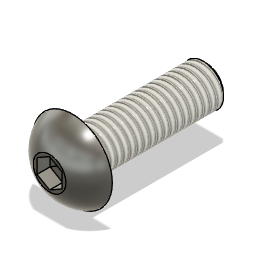
Microstat  Assembly v9 (Autodesk Fusion 360 archive; units mm, degrees)
design "Broached Hexagon Socket Button Head Cap Screw ASME B18.3.4M - M5 x 0.8 x 16 Steel Grade 2 Plain"
description: Broached Hexagon Socket Button Head Cap Screw ASME B18.3.4M - M5 x 0.8 x 16
part number: BHSBHCS ASME B18.3.4M - M5 x 0.8 x 16 Steel Grade 2 Plain
Autodesk Fusion 360 part; units mm, degrees
sketch "Sketch1" plane through (0, 0, 0) normal (0, 1, 0) x (1, 0, 0)
  line L0 (-2.5, 0) -> (-2.5, 16)
  line L1 (-2.5, 16) -> (0, 16)
  line L2 (0, 16) -> (0, -2.75)
  line L3 (-2.5, 0) -> (-4.75, 0)
  line L4 (0, -2.75) -> (-1.95, -2.75)
  arc A0 (-4.75, 0) -> (-1.95, -2.75) centre (0, 2.0359) ccw
  dimension "d9" = 5
  dimension "d66" = 9.5
  dimension "d98" = 3.9
  dimension "d105" = 2.75
  dimension "d106" = 16
  constraint perpendicular L0 L1
  constraint perpendicular L0 L3
  constraint coincident origin L3
  constraint vertical L0
  constraint vertical L2
  constraint coincident origin L2
  constraint perpendicular L2 L4
  constraint coincident L2 A0.centre
  measures "d105" distance of L3 L4
  measures "d106" distance of origin L1
revolve "Revolve1" add sketch "Sketch1" angle 360 about axis through (0, 0, -16) along (0, 0, 1)
ref_plane "WorkPlane1" through (0, 0, 2.75) normal (0, 0, 1) x (1, 0, 0)
sketch "Sketch6" plane through (0, 0, 2.75) normal (0, 0, 1) x (1, 0, 0)
  line L0 (-1.5, 0) -> (1.5, 0) construction
  line L1 (0, 0) -> (-1.5, 0.866)
  line L2 (-1.5, -0.866) -> (-1.5, 0.866)
  line L3 (-1.5, -0.866) -> (0, 0)
  dimension "d91" = 150
  dimension "d107" = 3
  constraint horizontal L0
  constraint midpoint L1.start L0
  constraint coincident L1.start L3.end
  constraint perpendicular L0 L2
  constraint midpoint L0.start L2
  constraint coincident L1.end L2.end
  measures "d91" angle of L0 L1
  measures "d107" distance of L0.end L2
extrude "Extrude1" cut sketch "Sketch6" against normal blind 1.56
pattern_circular "C-Pattern1" count 6 over 360 about axis through (0, 0, 1.75) along (0, 0, 1) of "Extrude1"
extrude "Extrude2" cut 1 faces at (0, -0.5774, 1.19) along direction (0, 0, -1) blind 1.56 draft -85
fillet "Fillet5" radius 0.2 1 edges at (-2.3308, 0.904, 0)
thread "Thread5" "ANSI Metric M Profile 5.0 M5x0.8 M5x0.8 4g6g" major diameter 4.901 minor diameter 4.007 pitch 0.8 angle 60 resizes the face on face at (-2.4876, 0.2489, -10.7333) from (0, 0, -1.6) to (0, 0, -16)
sketch "Sketch5" plane through (0, 0, 0) normal (0, 1, 0) x (1, 0, 0)
  line L0 (0, 16) -> (0, -2.75)
  line L1 (0, 16) -> (-2.55, 16)
  line L2 (-2.55, 16) -> (-2.55, 15.5092)
  line L3 (-2.55, 15.5092) -> (-2.0092, 16)
  dimension "d108" = 0.4908
  dimension "d109" = 2.0092
  dimension "d110" = 2.55
  constraint coincident L0.start L1.start
  constraint perpendicular L1 L2
  constraint coincident L1 L3.end
  measures "d108" distance of L1 L2.end
  measures "d109" distance of L0 L3.end
  measures "d110" distance of L0 L2
revolve "Revolve2" cut sketch "Sketch5" angle 360 about axis through (0, 0, -16) along (0, 0, 1)
equation "d9 = adsk_nomdia"
equation "adsk_nomlen = 16.00 mm"
equation "adsk_headh = 2.75 mm"
equation "adsk_headdia = 9.50 mm"
equation "adsk_nomdia = 5.00 mm"
equation "adsk_philwidth = 3.00 mm"
equation "d31 = -adsk_phildepth"
equation "adsk_phildepth = 1.56 mm"
equation "d66 = adsk_headdia"
equation "d71 = adsk_headh"
equation "d76 = -adsk_phildepth"
equation "adsk_thrlen = 14.40 mm"
equation "adsk_endpointdia = 4.01848 mm"
equation "adsk_startlen = 0.49076 mm"
equation "d98 = adsk_philwidth * 1.3"
equation "adsk_midfillet = 0.20 mm"
equation "d104 = adsk_midfillet"
equation "d105 = adsk_headh"
equation "d106 = adsk_nomlen"
equation "d107 = adsk_philwidth"
equation "d108 = adsk_startlen"
equation "d109 = adsk_endpointdia / 2"
equation "d110 = adsk_nomdia * 0.51"
equation "d116 = min(adsk_thrlen; adsk_nomlen - adsk_midfillet - 0.001 mm)"

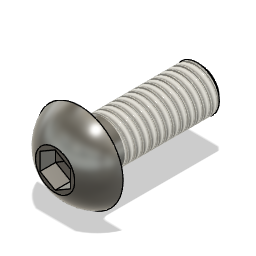
design "Hexagon Socket Button Head Screw ISO 7380-1 - M3 x 8 Steel 4.6 Plain"
description: Hexagon Socket Button Head Screw ISO 7380-1 - M3 x 8
part number: ISO 7380-1 - M3 x 8 Steel 4.6 Plain
Autodesk Fusion 360 part; units mm, degrees
sketch "Sketch1" plane through (0, 0, 0) normal (0, 1, 0) x (1, 0, 0)
  line L0 (-1.5, 0) -> (-1.5, 8)
  line L1 (-1.5, 8) -> (0, 8)
  line L2 (0, 8) -> (0, -1.65)
  line L3 (-1.5, 0) -> (-2.85, 0)
  line L4 (0, -1.65) -> (-1.3, -1.65)
  arc A0 (-2.85, 0) -> (-1.3, -1.65) centre (0, 1.1242) ccw
  dimension "d9" = 3
  dimension "d66" = 5.7
  dimension "d98" = 2.6
  dimension "d105" = 1.65
  dimension "d106" = 8
  constraint perpendicular L0 L1
  constraint perpendicular L0 L3
  constraint coincident origin L3
  constraint vertical L0
  constraint vertical L2
  constraint coincident origin L2
  constraint perpendicular L2 L4
  constraint coincident L2 A0.centre
  measures "d105" distance of L3 L4
  measures "d106" distance of origin L1
revolve "Revolve1" add sketch "Sketch1" angle 360 about axis through (0, 0, -8) along (0, 0, 1)
ref_plane "WorkPlane1" through (0, 0, 1.65) normal (0, 0, 1) x (1, 0, 0)
sketch "Sketch6" plane through (0, 0, 1.65) normal (0, 0, 1) x (1, 0, 0)
  line L0 (-1, 0) -> (1, 0) construction
  line L1 (0, 0) -> (-1, 0.5774)
  line L2 (-1, -0.5774) -> (-1, 0.5774)
  line L3 (-1, -0.5774) -> (0, 0)
  dimension "d91" = 150
  dimension "d107" = 2
  constraint horizontal L0
  constraint midpoint L1.start L0
  constraint coincident L1.start L3.end
  constraint perpendicular L0 L2
  constraint midpoint L0.start L2
  constraint coincident L1.end L2.end
  measures "d91" angle of L0 L1
  measures "d107" distance of L0.end L2
extrude "Extrude1" cut sketch "Sketch6" against normal blind 1.04
pattern_circular "C-Pattern1" count 6 over 360 about axis through (0, 0, 1.75) along (0, 0, 1) of "Extrude1"
extrude "Extrude2" cut 1 faces at (-0.3333, 0.1925, 0.61) along direction (0, 0, -1) blind 1.04 draft -85
fillet "Fillet5" radius 0.3 1 edges at (-1.3985, 0.5424, 0)
thread "Thread5" "ISO Metric profile 3.0 M3x0.5 M3x0.5 6g" major diameter 2.927 minor diameter 2.3555 pitch 0.5 angle 60 resizes the face on face at (-1.4981, 0.0748, -5.4333) from (0, 0, -1.5) to (0, 0, -8)
sketch "Sketch5" plane through (0, 0, 0) normal (0, 1, 0) x (1, 0, 0)
  line L0 (0, 8) -> (0, -1.65)
  line L1 (0, 8) -> (-1.53, 8)
  line L2 (-1.53, 8) -> (-1.53, 7.6933)
  line L3 (-1.53, 7.6933) -> (-1.1933, 8)
  dimension "d108" = 0.3067
  dimension "d109" = 1.1933
  dimension "d110" = 1.53
  constraint coincident L0.start L1.start
  constraint perpendicular L1 L2
  constraint coincident L1 L3.end
  measures "d108" distance of L1 L2.end
  measures "d109" distance of L0 L3.end
  measures "d110" distance of L0 L2
revolve "Revolve2" cut sketch "Sketch5" angle 360 about axis through (0, 0, -8) along (0, 0, 1)
equation "d9 = adsk_nomdia"
equation "adsk_nomlen = 8.00 mm"
equation "adsk_headh = 1.65 mm"
equation "adsk_headdia = 5.70 mm"
equation "adsk_nomdia = 3.00 mm"
equation "adsk_philwidth = 2.00 mm"
equation "d31 = -adsk_phildepth"
equation "adsk_phildepth = 1.04 mm"
equation "d66 = adsk_headdia"
equation "d71 = adsk_headh"
equation "d76 = -adsk_phildepth"
equation "adsk_thrlen = 6.50 mm"
equation "adsk_endpointdia = 2.38655 mm"
equation "adsk_startlen = 0.306725 mm"
equation "d98 = adsk_philwidth * 1.3"
equation "adsk_midfillet = 0.30 mm"
equation "d104 = adsk_midfillet"
equation "d105 = adsk_headh"
equation "d106 = adsk_nomlen"
equation "d107 = adsk_philwidth"
equation "d108 = adsk_startlen"
equation "d109 = adsk_endpointdia / 2"
equation "d110 = adsk_nomdia * 0.51"
equation "d116 = min(adsk_thrlen; adsk_nomlen - adsk_midfillet - 0.001 mm)"

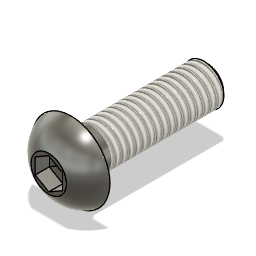
design "Hexagon Socket Button Head Screw ISO 7380-1 - M3 x 10 Steel 4.6 Plain"
description: Hexagon Socket Button Head Screw ISO 7380-1 - M3 x 10
part number: ISO 7380-1 - M3 x 10 Steel 4.6 Plain
Autodesk Fusion 360 part; units mm, degrees
sketch "Sketch1" plane through (0, 0, 0) normal (0, 1, 0) x (1, 0, 0)
  line L0 (-1.5, 0) -> (-1.5, 10)
  line L1 (-1.5, 10) -> (0, 10)
  line L2 (0, 10) -> (0, -1.65)
  line L3 (-1.5, 0) -> (-2.85, 0)
  line L4 (0, -1.65) -> (-1.3, -1.65)
  arc A0 (-2.85, 0) -> (-1.3, -1.65) centre (0, 1.1242) ccw
  dimension "d9" = 3
  dimension "d66" = 5.7
  dimension "d98" = 2.6
  dimension "d105" = 1.65
  dimension "d106" = 10
  constraint perpendicular L0 L1
  constraint perpendicular L0 L3
  constraint coincident origin L3
  constraint vertical L0
  constraint vertical L2
  constraint coincident origin L2
  constraint perpendicular L2 L4
  constraint coincident L2 A0.centre
  measures "d105" distance of L3 L4
  measures "d106" distance of origin L1
revolve "Revolve1" add sketch "Sketch1" angle 360 about axis through (0, 0, -10) along (0, 0, 1)
ref_plane "WorkPlane1" through (0, 0, 1.65) normal (0, 0, 1) x (1, 0, 0)
sketch "Sketch6" plane through (0, 0, 1.65) normal (0, 0, 1) x (1, 0, 0)
  line L0 (-1, 0) -> (1, 0) construction
  line L1 (0, 0) -> (-1, 0.5774)
  line L2 (-1, -0.5774) -> (-1, 0.5774)
  line L3 (-1, -0.5774) -> (0, 0)
  dimension "d91" = 150
  dimension "d107" = 2
  constraint horizontal L0
  constraint midpoint L1.start L0
  constraint coincident L1.start L3.end
  constraint perpendicular L0 L2
  constraint midpoint L0.start L2
  constraint coincident L1.end L2.end
  measures "d91" angle of L0 L1
  measures "d107" distance of L0.end L2
extrude "Extrude1" cut sketch "Sketch6" against normal blind 1.04
pattern_circular "C-Pattern1" count 6 over 360 about axis through (0, 0, 1.75) along (0, 0, 1) of "Extrude1"
extrude "Extrude2" cut 1 faces at (0, 0, 0.61) along direction (0, 0, -1) blind 1.04 draft -85
fillet "Fillet5" radius 0.3 1 edges at (-1.3985, 0.5424, 0)
thread "Thread5" "ISO Metric profile 3.0 M3x0.5 M3x0.5 6g" major diameter 2.927 minor diameter 2.3555 pitch 0.5 angle 60 resizes the face on face at (-1.4981, 0.0748, -6.7667) from (0, 0, -1.5) to (0, 0, -10)
sketch "Sketch5" plane through (0, 0, 0) normal (0, 1, 0) x (1, 0, 0)
  line L0 (0, 10) -> (0, -1.65)
  line L1 (0, 10) -> (-1.53, 10)
  line L2 (-1.53, 10) -> (-1.53, 9.6933)
  line L3 (-1.53, 9.6933) -> (-1.1933, 10)
  dimension "d108" = 0.3067
  dimension "d109" = 1.1933
  dimension "d110" = 1.53
  constraint coincident L0.start L1.start
  constraint perpendicular L1 L2
  constraint coincident L1 L3.end
  measures "d108" distance of L1 L2.end
  measures "d109" distance of L0 L3.end
  measures "d110" distance of L0 L2
revolve "Revolve2" cut sketch "Sketch5" angle 360 about axis through (0, 0, -10) along (0, 0, 1)
equation "d9 = adsk_nomdia"
equation "adsk_nomlen = 10.00 mm"
equation "adsk_headh = 1.65 mm"
equation "adsk_headdia = 5.70 mm"
equation "adsk_nomdia = 3.00 mm"
equation "adsk_philwidth = 2.00 mm"
equation "d31 = -adsk_phildepth"
equation "adsk_phildepth = 1.04 mm"
equation "d66 = adsk_headdia"
equation "d71 = adsk_headh"
equation "d76 = -adsk_phildepth"
equation "adsk_thrlen = 8.50 mm"
equation "adsk_endpointdia = 2.38655 mm"
equation "adsk_startlen = 0.306725 mm"
equation "d98 = adsk_philwidth * 1.3"
equation "adsk_midfillet = 0.30 mm"
equation "d104 = adsk_midfillet"
equation "d105 = adsk_headh"
equation "d106 = adsk_nomlen"
equation "d107 = adsk_philwidth"
equation "d108 = adsk_startlen"
equation "d109 = adsk_endpointdia / 2"
equation "d110 = adsk_nomdia * 0.51"
equation "d116 = min(adsk_thrlen; adsk_nomlen - adsk_midfillet - 0.001 mm)"

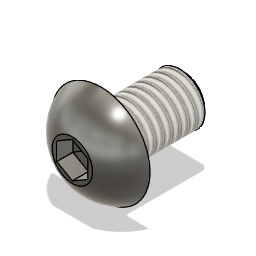
design "Broached Hexagon Socket Button Head Cap Screw ASME B18.3.4M - M5 x 0.8 x 8 Steel Grade 2 Plain"
description: Broached Hexagon Socket Button Head Cap Screw ASME B18.3.4M - M5 x 0.8 x 8
part number: BHSBHCS ASME B18.3.4M - M5 x 0.8 x 8 Steel Grade 2 Plain
Autodesk Fusion 360 part; units mm, degrees
sketch "Sketch1" plane through (0, 0, 0) normal (0, 1, 0) x (1, 0, 0)
  line L0 (-2.5, 0) -> (-2.5, 8)
  line L1 (-2.5, 8) -> (0, 8)
  line L2 (0, 8) -> (0, -2.75)
  line L3 (-2.5, 0) -> (-4.75, 0)
  line L4 (0, -2.75) -> (-1.95, -2.75)
  arc A0 (-4.75, 0) -> (-1.95, -2.75) centre (0, 2.0359) ccw
  dimension "d9" = 5
  dimension "d66" = 9.5
  dimension "d98" = 3.9
  dimension "d105" = 2.75
  dimension "d106" = 8
  constraint perpendicular L0 L1
  constraint perpendicular L0 L3
  constraint coincident origin L3
  constraint vertical L0
  constraint vertical L2
  constraint coincident origin L2
  constraint perpendicular L2 L4
  constraint coincident L2 A0.centre
  measures "d105" distance of L3 L4
  measures "d106" distance of origin L1
revolve "Revolve1" add sketch "Sketch1" angle 360 about axis through (0, 0, -8) along (0, 0, 1)
ref_plane "WorkPlane1" through (0, 0, 2.75) normal (0, 0, 1) x (1, 0, 0)
sketch "Sketch6" plane through (0, 0, 2.75) normal (0, 0, 1) x (1, 0, 0)
  line L0 (-1.5, 0) -> (1.5, 0) construction
  line L1 (0, 0) -> (-1.5, 0.866)
  line L2 (-1.5, -0.866) -> (-1.5, 0.866)
  line L3 (-1.5, -0.866) -> (0, 0)
  dimension "d91" = 150
  dimension "d107" = 3
  constraint horizontal L0
  constraint midpoint L1.start L0
  constraint coincident L1.start L3.end
  constraint perpendicular L0 L2
  constraint midpoint L0.start L2
  constraint coincident L1.end L2.end
  measures "d91" angle of L0 L1
  measures "d107" distance of L0.end L2
extrude "Extrude1" cut sketch "Sketch6" against normal blind 1.56
pattern_circular "C-Pattern1" count 6 over 360 about axis through (0, 0, 1.75) along (0, 0, 1) of "Extrude1"
extrude "Extrude2" cut 1 faces at (0.5, 0.2887, 1.19) along direction (0, 0, -1) blind 1.56 draft -85
fillet "Fillet5" radius 0.2 1 edges at (-2.3308, 0.904, 0)
thread "Thread5" "ANSI Metric M Profile 5.0 M5x0.8 M5x0.8 4g6g" major diameter 4.901 minor diameter 4.007 pitch 0.8 angle 60 resizes the face on face at (-2.4876, 0.2489, -5.4) from (0, 0, -1.6) to (0, 0, -8)
sketch "Sketch5" plane through (0, 0, 0) normal (0, 1, 0) x (1, 0, 0)
  line L0 (0, 8) -> (0, -2.75)
  line L1 (0, 8) -> (-2.55, 8)
  line L2 (-2.55, 8) -> (-2.55, 7.5092)
  line L3 (-2.55, 7.5092) -> (-2.0092, 8)
  dimension "d108" = 0.4908
  dimension "d109" = 2.0092
  dimension "d110" = 2.55
  constraint coincident L0.start L1.start
  constraint perpendicular L1 L2
  constraint coincident L1 L3.end
  measures "d108" distance of L1 L2.end
  measures "d109" distance of L0 L3.end
  measures "d110" distance of L0 L2
revolve "Revolve2" cut sketch "Sketch5" angle 360 about axis through (0, 0, -8) along (0, 0, 1)
equation "d9 = adsk_nomdia"
equation "adsk_nomlen = 8.00 mm"
equation "adsk_headh = 2.75 mm"
equation "adsk_headdia = 9.50 mm"
equation "adsk_nomdia = 5.00 mm"
equation "adsk_philwidth = 3.00 mm"
equation "d31 = -adsk_phildepth"
equation "adsk_phildepth = 1.56 mm"
equation "d66 = adsk_headdia"
equation "d71 = adsk_headh"
equation "d76 = -adsk_phildepth"
equation "adsk_thrlen = 6.40 mm"
equation "adsk_endpointdia = 4.01848 mm"
equation "adsk_startlen = 0.49076 mm"
equation "d98 = adsk_philwidth * 1.3"
equation "adsk_midfillet = 0.20 mm"
equation "d104 = adsk_midfillet"
equation "d105 = adsk_headh"
equation "d106 = adsk_nomlen"
equation "d107 = adsk_philwidth"
equation "d108 = adsk_startlen"
equation "d109 = adsk_endpointdia / 2"
equation "d110 = adsk_nomdia * 0.51"
equation "d116 = min(adsk_thrlen; adsk_nomlen - adsk_midfillet - 0.001 mm)"

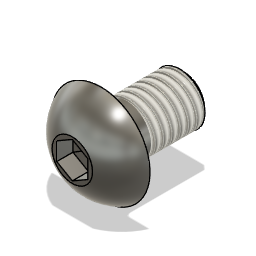
design "Hexagon Socket Button Head Screw ISO 7380-1 - M5 x 8 Steel 4.6 Plain"
description: Hexagon Socket Button Head Screw ISO 7380-1 - M5 x 8
part number: ISO 7380-1 - M5 x 8 Steel 4.6 Plain
Autodesk Fusion 360 part; units mm, degrees
sketch "Sketch1" plane through (0, 0, 0) normal (0, 1, 0) x (1, 0, 0)
  line L0 (-2.5, 0) -> (-2.5, 8)
  line L1 (-2.5, 8) -> (0, 8)
  line L2 (0, 8) -> (0, -2.75)
  line L3 (-2.5, 0) -> (-4.75, 0)
  line L4 (0, -2.75) -> (-1.95, -2.75)
  arc A0 (-4.75, 0) -> (-1.95, -2.75) centre (0, 2.0359) ccw
  dimension "d9" = 5
  dimension "d66" = 9.5
  dimension "d98" = 3.9
  dimension "d105" = 2.75
  dimension "d106" = 8
  constraint perpendicular L0 L1
  constraint perpendicular L0 L3
  constraint coincident origin L3
  constraint vertical L0
  constraint vertical L2
  constraint coincident origin L2
  constraint perpendicular L2 L4
  constraint coincident L2 A0.centre
  measures "d105" distance of L3 L4
  measures "d106" distance of origin L1
revolve "Revolve1" add sketch "Sketch1" angle 360 about axis through (0, 0, -8) along (0, 0, 1)
ref_plane "WorkPlane1" through (0, 0, 2.75) normal (0, 0, 1) x (1, 0, 0)
sketch "Sketch6" plane through (0, 0, 2.75) normal (0, 0, 1) x (1, 0, 0)
  line L0 (-1.5, 0) -> (1.5, 0) construction
  line L1 (0, 0) -> (-1.5, 0.866)
  line L2 (-1.5, -0.866) -> (-1.5, 0.866)
  line L3 (-1.5, -0.866) -> (0, 0)
  dimension "d91" = 150
  dimension "d107" = 3
  constraint horizontal L0
  constraint midpoint L1.start L0
  constraint coincident L1.start L3.end
  constraint perpendicular L0 L2
  constraint midpoint L0.start L2
  constraint coincident L1.end L2.end
  measures "d91" angle of L0 L1
  measures "d107" distance of L0.end L2
extrude "Extrude1" cut sketch "Sketch6" against normal blind 1.56
pattern_circular "C-Pattern1" count 6 over 360 about axis through (0, 0, 1.75) along (0, 0, 1) of "Extrude1"
extrude "Extrude2" cut 1 faces at (0.5, 0.2887, 1.19) along direction (0, 0, -1) blind 1.56 draft -85
fillet "Fillet5" radius 0.45 1 edges at (-2.3308, 0.904, 0)
thread "Thread5" "ISO Metric profile 5.0 M5x0.8 M5x0.8 6g" major diameter 4.901 minor diameter 3.9895 pitch 0.8 angle 60 resizes the face on face at (-2.4876, 0.2489, -5.4833) from (0, 0, -2.4) to (0, 0, -8)
sketch "Sketch5" plane through (0, 0, 0) normal (0, 1, 0) x (1, 0, 0)
  line L0 (0, 8) -> (0, -2.75)
  line L1 (0, 8) -> (-2.55, 8)
  line L2 (-2.55, 8) -> (-2.55, 7.5092)
  line L3 (-2.55, 7.5092) -> (-2.0092, 8)
  dimension "d108" = 0.4908
  dimension "d109" = 2.0092
  dimension "d110" = 2.55
  constraint coincident L0.start L1.start
  constraint perpendicular L1 L2
  constraint coincident L1 L3.end
  measures "d108" distance of L1 L2.end
  measures "d109" distance of L0 L3.end
  measures "d110" distance of L0 L2
revolve "Revolve2" cut sketch "Sketch5" angle 360 about axis through (0, 0, -8) along (0, 0, 1)
equation "d9 = adsk_nomdia"
equation "adsk_nomlen = 8.00 mm"
equation "adsk_headh = 2.75 mm"
equation "adsk_headdia = 9.50 mm"
equation "adsk_nomdia = 5.00 mm"
equation "adsk_philwidth = 3.00 mm"
equation "d31 = -adsk_phildepth"
equation "adsk_phildepth = 1.56 mm"
equation "d66 = adsk_headdia"
equation "d71 = adsk_headh"
equation "d76 = -adsk_phildepth"
equation "adsk_thrlen = 5.60 mm"
equation "adsk_endpointdia = 4.01848 mm"
equation "adsk_startlen = 0.49076 mm"
equation "d98 = adsk_philwidth * 1.3"
equation "adsk_midfillet = 0.45 mm"
equation "d104 = adsk_midfillet"
equation "d105 = adsk_headh"
equation "d106 = adsk_nomlen"
equation "d107 = adsk_philwidth"
equation "d108 = adsk_startlen"
equation "d109 = adsk_endpointdia / 2"
equation "d110 = adsk_nomdia * 0.51"
equation "d116 = min(adsk_thrlen; adsk_nomlen - adsk_midfillet - 0.001 mm)"

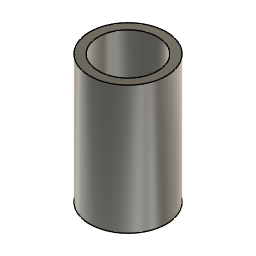
design "inner_payload_rod"
Autodesk Fusion 360 part; units mm, degrees
sketch "Sketch1" plane through (0, 0, 0) normal (0, 0, 1) x (1, 0, 0)
  circle A0 centre (0, 0) radius 7.75
  dimension "d1" = 15.5
  constraint coincident A0.centre origin
  measures "d1" diameter of A0
extrude "Extrude1" add sketch "Sketch1" along normal blind 26
sketch "Sketch2" plane through (0, 0, 26) normal (0, 0, 1) x (-1, 0, 0)
  circle A0 centre (0, 0) radius 7.75
  circle A1 centre (0, 0) radius 6
  dimension "d4" = 12
  constraint concentric A0 A1
  measures "d4" diameter of A1
extrude "Extrude2" cut sketch "Sketch2" against normal blind 26 contours A1

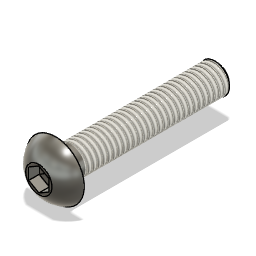
design "Hexagon Socket Button Head Screw ISO 7380-1 - M3 x 16 Steel 4.6 Plain"
description: Hexagon Socket Button Head Screw ISO 7380-1 - M3 x 16
part number: ISO 7380-1 - M3 x 16 Steel 4.6 Plain
Autodesk Fusion 360 part; units mm, degrees
sketch "Sketch1" plane through (0, 0, 0) normal (0, 1, 0) x (1, 0, 0)
  line L0 (-1.5, 0) -> (-1.5, 16)
  line L1 (-1.5, 16) -> (0, 16)
  line L2 (0, 16) -> (0, -1.65)
  line L3 (-1.5, 0) -> (-2.85, 0)
  line L4 (0, -1.65) -> (-1.3, -1.65)
  arc A0 (-2.85, 0) -> (-1.3, -1.65) centre (0, 1.1242) ccw
  dimension "d9" = 3
  dimension "d66" = 5.7
  dimension "d98" = 2.6
  dimension "d105" = 1.65
  dimension "d106" = 16
  constraint perpendicular L0 L1
  constraint perpendicular L0 L3
  constraint coincident origin L3
  constraint vertical L0
  constraint vertical L2
  constraint coincident origin L2
  constraint perpendicular L2 L4
  constraint coincident L2 A0.centre
  measures "d105" distance of L3 L4
  measures "d106" distance of origin L1
revolve "Revolve1" add sketch "Sketch1" angle 360 about axis through (0, 0, -16) along (0, 0, 1)
ref_plane "WorkPlane1" through (0, 0, 1.65) normal (0, 0, 1) x (1, 0, 0)
sketch "Sketch6" plane through (0, 0, 1.65) normal (0, 0, 1) x (1, 0, 0)
  line L0 (-1, 0) -> (1, 0) construction
  line L1 (0, 0) -> (-1, 0.5774)
  line L2 (-1, -0.5774) -> (-1, 0.5774)
  line L3 (-1, -0.5774) -> (0, 0)
  dimension "d91" = 150
  dimension "d107" = 2
  constraint horizontal L0
  constraint midpoint L1.start L0
  constraint coincident L1.start L3.end
  constraint perpendicular L0 L2
  constraint midpoint L0.start L2
  constraint coincident L1.end L2.end
  measures "d91" angle of L0 L1
  measures "d107" distance of L0.end L2
extrude "Extrude1" cut sketch "Sketch6" against normal blind 1.04
pattern_circular "C-Pattern1" count 6 over 360 about axis through (0, 0, 1.75) along (0, 0, 1) of "Extrude1"
extrude "Extrude2" cut 1 faces at (-0.3333, 0.1925, 0.61) along direction (0, 0, -1) blind 1.04 draft -85
fillet "Fillet5" radius 0.3 1 edges at (-1.3985, 0.5424, 0)
thread "Thread5" "ISO Metric profile 3.0 M3x0.5 M3x0.5 6g" major diameter 2.927 minor diameter 2.3555 pitch 0.5 angle 60 resizes the face on face at (-1.4981, 0.0748, -10.7667) from (0, 0, -1.5) to (0, 0, -16)
sketch "Sketch5" plane through (0, 0, 0) normal (0, 1, 0) x (1, 0, 0)
  line L0 (0, 16) -> (0, -1.65)
  line L1 (0, 16) -> (-1.53, 16)
  line L2 (-1.53, 16) -> (-1.53, 15.6933)
  line L3 (-1.53, 15.6933) -> (-1.1933, 16)
  dimension "d108" = 0.3067
  dimension "d109" = 1.1933
  dimension "d110" = 1.53
  constraint coincident L0.start L1.start
  constraint perpendicular L1 L2
  constraint coincident L1 L3.end
  measures "d108" distance of L1 L2.end
  measures "d109" distance of L0 L3.end
  measures "d110" distance of L0 L2
revolve "Revolve2" cut sketch "Sketch5" angle 360 about axis through (0, 0, -16) along (0, 0, 1)
equation "d9 = adsk_nomdia"
equation "adsk_nomlen = 16.00 mm"
equation "adsk_headh = 1.65 mm"
equation "adsk_headdia = 5.70 mm"
equation "adsk_nomdia = 3.00 mm"
equation "adsk_philwidth = 2.00 mm"
equation "d31 = -adsk_phildepth"
equation "adsk_phildepth = 1.04 mm"
equation "d66 = adsk_headdia"
equation "d71 = adsk_headh"
equation "d76 = -adsk_phildepth"
equation "adsk_thrlen = 14.50 mm"
equation "adsk_endpointdia = 2.38655 mm"
equation "adsk_startlen = 0.306725 mm"
equation "d98 = adsk_philwidth * 1.3"
equation "adsk_midfillet = 0.30 mm"
equation "d104 = adsk_midfillet"
equation "d105 = adsk_headh"
equation "d106 = adsk_nomlen"
equation "d107 = adsk_philwidth"
equation "d108 = adsk_startlen"
equation "d109 = adsk_endpointdia / 2"
equation "d110 = adsk_nomdia * 0.51"
equation "d116 = min(adsk_thrlen; adsk_nomlen - adsk_midfillet - 0.001 mm)"

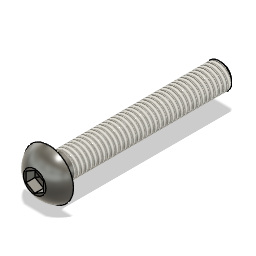
design "Hexagon Socket Button Head Screw ISO 7380-1 - M3 x 20 Steel 4.6 Plain"
description: Hexagon Socket Button Head Screw ISO 7380-1 - M3 x 20
part number: ISO 7380-1 - M3 x 20 Steel 4.6 Plain
Autodesk Fusion 360 part; units mm, degrees
sketch "Sketch1" plane through (0, 0, 0) normal (0, 1, 0) x (1, 0, 0)
  line L0 (-1.5, 0) -> (-1.5, 20)
  line L1 (-1.5, 20) -> (0, 20)
  line L2 (0, 20) -> (0, -1.65)
  line L3 (-1.5, 0) -> (-2.85, 0)
  line L4 (0, -1.65) -> (-1.3, -1.65)
  arc A0 (-2.85, 0) -> (-1.3, -1.65) centre (0, 1.1242) ccw
  dimension "d9" = 3
  dimension "d66" = 5.7
  dimension "d98" = 2.6
  dimension "d105" = 1.65
  dimension "d106" = 20
  constraint perpendicular L0 L1
  constraint perpendicular L0 L3
  constraint coincident origin L3
  constraint vertical L0
  constraint vertical L2
  constraint coincident origin L2
  constraint perpendicular L2 L4
  constraint coincident L2 A0.centre
  measures "d105" distance of L3 L4
  measures "d106" distance of origin L1
revolve "Revolve1" add sketch "Sketch1" angle 360 about axis through (0, 0, -20) along (0, 0, 1)
ref_plane "WorkPlane1" through (0, 0, 1.65) normal (0, 0, 1) x (1, 0, 0)
sketch "Sketch6" plane through (0, 0, 1.65) normal (0, 0, 1) x (1, 0, 0)
  line L0 (-1, 0) -> (1, 0) construction
  line L1 (0, 0) -> (-1, 0.5774)
  line L2 (-1, -0.5774) -> (-1, 0.5774)
  line L3 (-1, -0.5774) -> (0, 0)
  dimension "d91" = 150
  dimension "d107" = 2
  constraint horizontal L0
  constraint midpoint L1.start L0
  constraint coincident L1.start L3.end
  constraint perpendicular L0 L2
  constraint midpoint L0.start L2
  constraint coincident L1.end L2.end
  measures "d91" angle of L0 L1
  measures "d107" distance of L0.end L2
extrude "Extrude1" cut sketch "Sketch6" against normal blind 1.04
pattern_circular "C-Pattern1" count 6 over 360 about axis through (0, 0, 1.75) along (0, 0, 1) of "Extrude1"
extrude "Extrude2" cut 1 faces at (0, 0, 0.61) along direction (0, 0, -1) blind 1.04 draft -85
fillet "Fillet5" radius 0.3 1 edges at (-1.3985, 0.5424, 0)
thread "Thread5" "ISO Metric profile 3.0 M3x0.5 M3x0.5 6g" major diameter 2.927 minor diameter 2.3555 pitch 0.5 angle 60 resizes the face on face at (-1.4981, 0.0748, -13.4333) from (0, 0, -1.5) to (0, 0, -20)
sketch "Sketch5" plane through (0, 0, 0) normal (0, 1, 0) x (1, 0, 0)
  line L0 (0, 20) -> (0, -1.65)
  line L1 (0, 20) -> (-1.53, 20)
  line L2 (-1.53, 20) -> (-1.53, 19.6933)
  line L3 (-1.53, 19.6933) -> (-1.1933, 20)
  dimension "d108" = 0.3067
  dimension "d109" = 1.1933
  dimension "d110" = 1.53
  constraint coincident L0.start L1.start
  constraint perpendicular L1 L2
  constraint coincident L1 L3.end
  measures "d108" distance of L1 L2.end
  measures "d109" distance of L0 L3.end
  measures "d110" distance of L0 L2
revolve "Revolve2" cut sketch "Sketch5" angle 360 about axis through (0, 0, -20) along (0, 0, 1)
equation "d9 = adsk_nomdia"
equation "adsk_nomlen = 20.00 mm"
equation "adsk_headh = 1.65 mm"
equation "adsk_headdia = 5.70 mm"
equation "adsk_nomdia = 3.00 mm"
equation "adsk_philwidth = 2.00 mm"
equation "d31 = -adsk_phildepth"
equation "adsk_phildepth = 1.04 mm"
equation "d66 = adsk_headdia"
equation "d71 = adsk_headh"
equation "d76 = -adsk_phildepth"
equation "adsk_thrlen = 18.50 mm"
equation "adsk_endpointdia = 2.38655 mm"
equation "adsk_startlen = 0.306725 mm"
equation "d98 = adsk_philwidth * 1.3"
equation "adsk_midfillet = 0.30 mm"
equation "d104 = adsk_midfillet"
equation "d105 = adsk_headh"
equation "d106 = adsk_nomlen"
equation "d107 = adsk_philwidth"
equation "d108 = adsk_startlen"
equation "d109 = adsk_endpointdia / 2"
equation "d110 = adsk_nomdia * 0.51"
equation "d116 = min(adsk_thrlen; adsk_nomlen - adsk_midfillet - 0.001 mm)"

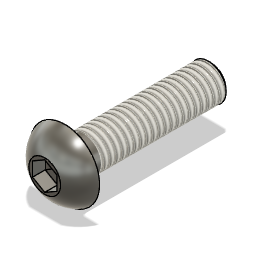
design "Hexagon Socket Button Head Screw ISO 7380-1 - M3 x 12 Steel 4.6 Plain"
description: Hexagon Socket Button Head Screw ISO 7380-1 - M3 x 12
part number: ISO 7380-1 - M3 x 12 Steel 4.6 Plain
Autodesk Fusion 360 part; units mm, degrees
sketch "Sketch1" plane through (0, 0, 0) normal (0, 1, 0) x (1, 0, 0)
  line L0 (-1.5, 0) -> (-1.5, 12)
  line L1 (-1.5, 12) -> (0, 12)
  line L2 (0, 12) -> (0, -1.65)
  line L3 (-1.5, 0) -> (-2.85, 0)
  line L4 (0, -1.65) -> (-1.3, -1.65)
  arc A0 (-2.85, 0) -> (-1.3, -1.65) centre (0, 1.1242) ccw
  dimension "d9" = 3
  dimension "d66" = 5.7
  dimension "d98" = 2.6
  dimension "d105" = 1.65
  dimension "d106" = 12
  constraint perpendicular L0 L1
  constraint perpendicular L0 L3
  constraint coincident origin L3
  constraint vertical L0
  constraint vertical L2
  constraint coincident origin L2
  constraint perpendicular L2 L4
  constraint coincident L2 A0.centre
  measures "d105" distance of L3 L4
  measures "d106" distance of origin L1
revolve "Revolve1" add sketch "Sketch1" angle 360 about axis through (0, 0, -12) along (0, 0, 1)
ref_plane "WorkPlane1" through (0, 0, 1.65) normal (0, 0, 1) x (1, 0, 0)
sketch "Sketch6" plane through (0, 0, 1.65) normal (0, 0, 1) x (1, 0, 0)
  line L0 (-1, 0) -> (1, 0) construction
  line L1 (0, 0) -> (-1, 0.5774)
  line L2 (-1, -0.5774) -> (-1, 0.5774)
  line L3 (-1, -0.5774) -> (0, 0)
  dimension "d91" = 150
  dimension "d107" = 2
  constraint horizontal L0
  constraint midpoint L1.start L0
  constraint coincident L1.start L3.end
  constraint perpendicular L0 L2
  constraint midpoint L0.start L2
  constraint coincident L1.end L2.end
  measures "d91" angle of L0 L1
  measures "d107" distance of L0.end L2
extrude "Extrude1" cut sketch "Sketch6" against normal blind 1.04
pattern_circular "C-Pattern1" count 6 over 360 about axis through (0, 0, 1.75) along (0, 0, 1) of "Extrude1"
extrude "Extrude2" cut 1 faces at (0, 0, 0.61) along direction (0, 0, -1) blind 1.04 draft -85
fillet "Fillet5" radius 0.3 1 edges at (-1.3985, 0.5424, 0)
thread "Thread5" "ISO Metric profile 3.0 M3x0.5 M3x0.5 6g" major diameter 2.927 minor diameter 2.3555 pitch 0.5 angle 60 resizes the face on face at (-1.4981, 0.0748, -8.1) from (0, 0, -1.5) to (0, 0, -12)
sketch "Sketch5" plane through (0, 0, 0) normal (0, 1, 0) x (1, 0, 0)
  line L0 (0, 12) -> (0, -1.65)
  line L1 (0, 12) -> (-1.53, 12)
  line L2 (-1.53, 12) -> (-1.53, 11.6933)
  line L3 (-1.53, 11.6933) -> (-1.1933, 12)
  dimension "d108" = 0.3067
  dimension "d109" = 1.1933
  dimension "d110" = 1.53
  constraint coincident L0.start L1.start
  constraint perpendicular L1 L2
  constraint coincident L1 L3.end
  measures "d108" distance of L1 L2.end
  measures "d109" distance of L0 L3.end
  measures "d110" distance of L0 L2
revolve "Revolve2" cut sketch "Sketch5" angle 360 about axis through (0, 0, -12) along (0, 0, 1)
equation "d9 = adsk_nomdia"
equation "adsk_nomlen = 12.00 mm"
equation "adsk_headh = 1.65 mm"
equation "adsk_headdia = 5.70 mm"
equation "adsk_nomdia = 3.00 mm"
equation "adsk_philwidth = 2.00 mm"
equation "d31 = -adsk_phildepth"
equation "adsk_phildepth = 1.04 mm"
equation "d66 = adsk_headdia"
equation "d71 = adsk_headh"
equation "d76 = -adsk_phildepth"
equation "adsk_thrlen = 10.50 mm"
equation "adsk_endpointdia = 2.38655 mm"
equation "adsk_startlen = 0.306725 mm"
equation "d98 = adsk_philwidth * 1.3"
equation "adsk_midfillet = 0.30 mm"
equation "d104 = adsk_midfillet"
equation "d105 = adsk_headh"
equation "d106 = adsk_nomlen"
equation "d107 = adsk_philwidth"
equation "d108 = adsk_startlen"
equation "d109 = adsk_endpointdia / 2"
equation "d110 = adsk_nomdia * 0.51"
equation "d116 = min(adsk_thrlen; adsk_nomlen - adsk_midfillet - 0.001 mm)"

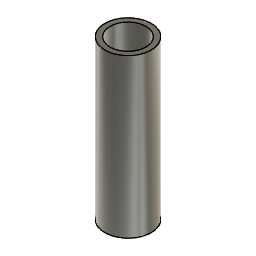
design "payload_chamber_rod"
Autodesk Fusion 360 part; units mm, degrees
sketch "Sketch1" plane through (0, 0, 0) normal (0, 0, 1) x (1, 0, 0)
  circle A0 centre (0, 0) radius 7.75
  dimension "d1" = 15.5
  constraint coincident A0.centre origin
  measures "d1" diameter of A0
extrude "Extrude1" add sketch "Sketch1" along normal blind 27.9
sketch "Sketch2" plane through (0, 0, 27.9) normal (0, 0, 1) x (-1, 0, 0)
  circle A0 centre (0, 0) radius 7.75
  circle A1 centre (0, 0) radius 6
  dimension "d4" = 12
  constraint concentric A0 A1
  measures "d4" diameter of A1
extrude "Extrude2" cut sketch "Sketch2" against normal blind 30 contours A1
extrude "Extrude3" add 1 faces at (7.1155, -0.6831, 27.9) along direction (0, 0, 1) blind 15
extrude "Extrude4" add 1 faces at (7.1155, -0.6831, 42.9) along direction (0, 0, 1) blind 10

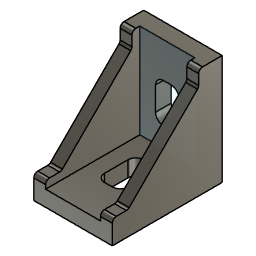
design "Angle Bracket v1"
Autodesk Fusion 360 part; units mm, degrees
sketch "Sketch1" plane through (0, 0, 0) normal (1, 0, 0) x (0, 1, 0)
  line L0 (0, 0) -> (28, 0)
  line L1 (28, 0) -> (28, 28)
  line L2 (28, 28) -> (22, 28)
  line L3 (22, 28) -> (22, 24)
  line L4 (0, 0) -> (0, 6)
  line L5 (0, 6) -> (4, 6)
  line L6 (4, 6) -> (22, 24)
  dimension "d1" = 28
  dimension "d2" = 28
  constraint coincident L0.start L4.start
  constraint horizontal L0
  constraint perpendicular L0 L1
  constraint perpendicular L1 L2
  constraint perpendicular L2 L3
  constraint perpendicular L0 L4
  constraint perpendicular L4 L5
  measures "d1" distance of L0.start L0.end
  measures "d2" distance of L0.end L1.end
extrude "Extrude1" add sketch "Sketch1" along normal blind 3
sketch "Sketch2" plane through (3, 0, 0) normal (1, 0, 0) x (0, 1, 0)
  line L0 (0, 0) -> (28, 0)
  line L1 (28, 0) -> (28, 28)
  line L2 (28, 28) -> (22, 28)
  line L3 (22, 28) -> (22, 24)
  line L4 (22, 24) -> (4, 6)
  line L5 (4, 6) -> (0, 6)
  line L6 (0, 6) -> (0, 0)
  line L7 (0, 0) -> (28, 0)
  line L8 (28, 0) -> (28, 4)
  line L9 (24, 4) -> (0, 4)
  line L10 (0, 4) -> (0, 0)
  line L11 (28, 28) -> (24, 28)
  line L12 (24, 28) -> (24, 4)
  line L13 (24, 0) -> (28, 0)
  line L14 (28, 0) -> (28, 28)
  dimension "d5" = 4
  dimension "d6" = 28
  constraint horizontal L7
  constraint vertical L8
  constraint horizontal L9
  constraint vertical L10
  constraint coincident L1 L8.end
  constraint coincident L0.start L6.end
  constraint horizontal L11
  constraint vertical L12
  constraint horizontal L13
  constraint vertical L14
  constraint coincident L1.end L2.start
  measures "d5" distance of L1.end L11.end
  measures "d6" distance of L1.end L0.end
extrude "Extrude2" add sketch "Sketch2" along normal blind 14 contours L0 L1 L2 L6 L7 L8 L9 L10 L11 L12 L13 L14
sketch "Sketch3" plane through (17, 0, 0) normal (1, 0, 0) x (0, 1, 0)
  line L0 (28, 0) -> (28, 28)
  line L1 (28, 28) -> (24, 28)
  line L2 (24, 28) -> (24, 4)
  line L3 (24, 4) -> (0, 4)
  line L4 (0, 4) -> (0, 0)
  line L5 (0, 0) -> (28, 0)
  line L6 (0, 0) -> (28, 0)
  line L7 (28, 28) -> (28, 0)
  line L8 (28, 28) -> (22, 28)
  line L9 (22, 28) -> (22, 24)
  line L10 (22, 24) -> (4, 6)
  line L11 (4, 6) -> (0, 6)
  line L12 (0, 6) -> (0, 0)
  constraint coincident L4.end L5.start
  constraint coincident L0.start L5.end
  constraint coincident L0.end L1.start
  constraint perpendicular L2 L8
  constraint perpendicular L8 L9
  constraint perpendicular L9 L11
  constraint perpendicular L6 L12
sketch "Sketch4" plane through (17, 0, 0) normal (1, 0, 0) x (0, 1, 0)
extrude "Extrude3" add sketch "Sketch3" along normal blind 3
sketch "Sketch5" plane through (0, 24, 0) normal (0, -1, 0) x (1, 0, 0)
  line L0 (3, 28) -> (3, 4)
  line L1 (3, 4) -> (17, 4)
  line L2 (17, 4) -> (17, 28)
  line L3 (17, 28) -> (3, 28)
fillet "Fillet1" radius 1 1 edges at (1.5, 22, 28)
fillet "Fillet2" radius 1 1 edges at (18.5, 22, 28)
fillet "Fillet3" radius 1 1 edges at (1.5, 0, 6)
fillet "Fillet4" radius 1 1 edges at (18.5, 0, 6)
fillet "Fillet5" radius 1 1 edges at (1.5, 4, 6)
fillet "Fillet6" radius 1 1 edges at (18.5, 4, 6)
fillet "Fillet7" radius 1 1 edges at (1.5, 22, 24)
fillet "Fillet8" radius 1 1 edges at (18.5, 22, 24)
sketch "Sketch6" plane through (0, 24, 0) normal (0, -1, 0) x (1, 0, 0)
  line L0 (11, 19) -> (9, 19)
  line L1 (7, 17) -> (7, 11)
  line L2 (9, 9) -> (11, 9)
  line L3 (13, 11) -> (13, 17)
  line L4 (13, 19) -> (7, 9) construction
  line L5 (7, 19) -> (13, 9) construction
  arc A0 (9, 19) -> (7, 17) centre (9, 17) ccw
  arc A1 (13, 17) -> (11, 19) centre (11, 17) ccw
  arc A2 (11, 9) -> (13, 11) centre (11, 11) ccw
  arc A3 (7, 11) -> (9, 9) centre (9, 11) ccw
  point P0 (10, 14)
  dimension "d27" = 6
  dimension "d28" = 10
  dimension "d29" = 2
  constraint horizontal L0
  constraint perpendicular L0 L1
  constraint parallel L0 L2
  constraint parallel L1 L3
  constraint coincident L4 P0
  constraint coincident L5 P0
  constraint coincident L5.start L0
  constraint coincident L5.start L1
  constraint tangent L0 A0
  constraint tangent L1 A0
  constraint coincident L4.start L3
  constraint coincident L4.start L0
  constraint tangent L3 A1
  constraint tangent L0 A1
  constraint equal A0 A1
  constraint coincident L5.end L3
  constraint coincident L5.end L2
  constraint tangent L3 A2
  constraint tangent L2 A2
  constraint equal A0 A2
  constraint coincident L4.end L1
  constraint coincident L4.end L2
  constraint tangent L1 A3
  constraint tangent L2 A3
  constraint equal A0 A3
  measures "d27" distance of L4.end L5.end
  measures "d28" distance of L5.start L4.end
  measures "d29" radius of A0
extrude "Extrude4" cut sketch "Sketch6" against normal blind 7
sketch "Sketch7" plane through (0, 0, 4) normal (0, 0, 1) x (-1, 0, 0)
  line L0 (-3, -24) -> (-3, 0)
  line L1 (-3, 0) -> (-17, 0)
  line L2 (-17, 0) -> (-17, -24)
  line L3 (-17, -24) -> (-3, -24)
  line L4 (-9, -9) -> (-11, -9)
  line L5 (-13, -11) -> (-13, -17)
  line L6 (-11, -19) -> (-9, -19)
  line L7 (-7, -17) -> (-7, -11)
  line L8 (-7, -9) -> (-13, -19) construction
  line L9 (-13, -9) -> (-7, -19) construction
  arc A0 (-9, -19) -> (-7, -17) centre (-9, -17) ccw
  arc A1 (-7, -11) -> (-9, -9) centre (-9, -11) ccw
  arc A2 (-13, -17) -> (-11, -19) centre (-11, -17) ccw
  arc A3 (-11, -9) -> (-13, -11) centre (-11, -11) ccw
  point P0 (-10, -14)
  dimension "d32" = 6
  dimension "d33" = 10
  dimension "d34" = 2
  constraint horizontal L4
  constraint perpendicular L4 L5
  constraint parallel L4 L6
  constraint parallel L5 L7
  constraint coincident L8 P0
  constraint coincident L9 P0
  constraint coincident L9.end L6
  constraint coincident L9.end L7
  constraint tangent L6 A0
  constraint tangent L7 A0
  constraint coincident L8.start L4
  constraint coincident L8.start L7
  constraint tangent L4 A1
  constraint tangent L7 A1
  constraint equal A0 A1
  constraint coincident L8.end L6
  constraint coincident L8.end L5
  constraint tangent L6 A2
  constraint tangent L5 A2
  constraint equal A0 A2
  constraint coincident L9.start L5
  constraint coincident L9.start L4
  constraint tangent L5 A3
  constraint tangent L4 A3
  constraint equal A0 A3
  measures "d32" distance of L8.end L9.end
  measures "d33" distance of L9.start L8.end
  measures "d34" radius of A0
extrude "Extrude5" cut sketch "Sketch7" against normal blind 4 contours L4 L5 L6 L7 A0 A1 A2 A3

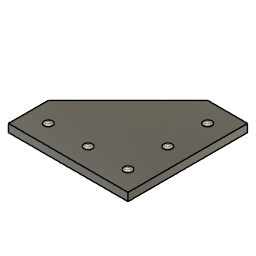
design "Bracket Plate v2"
Autodesk Fusion 360 part; units mm, degrees
sketch "Sketch1" plane through (0, 0, 0) normal (0, 0, 1) x (1, 0, 0)
  line L0 (0, 0) -> (60, 0)
  line L1 (60, 0) -> (60, 60)
  line L2 (60, 60) -> (40, 60)
  line L3 (0, 0) -> (0, 20)
  line L4 (0, 20) -> (40, 60)
  dimension "d1" = 60
  dimension "d2" = 60
  dimension "d3" = 20
  dimension "d4" = 20
  constraint coincident L0.start L3.start
  constraint horizontal L0
  constraint perpendicular L0 L1
  constraint perpendicular L1 L2
  constraint perpendicular L2 L3
  measures "d1" distance of L0.start L0.end
  measures "d2" distance of L0.end L1.end
  measures "d3" distance of L1.end L2.end
  measures "d4" distance of L0.start L3.end
extrude "Extrude1" add sketch "Sketch1" along normal blind 4
hole "Hole2" at (10, 10, 4) direction (0, 0, -1) diameter 4.234 depth 34 tip angle 180
thread "Thread2" "ANSI Metric M Profile 5.0 M5x0.8 6H" thread offset 0 thread depth 7.4
hole "Hole3" at (50, 10, 4) direction (0, 0, -1) diameter 4.234 depth 34 tip angle 180
thread "Thread3" "ANSI Metric M Profile 5.0 M5x0.8 6H" major diameter 5.12 minor diameter 4.234 pitch 0.8 angle 60 resizes the face on face at (50.2108, 12.1065, 2.6667)
hole "Hole4" at (50, 50, 4) direction (0, 0, -1) diameter 4.234 depth 34 tip angle 180
thread "Thread4" "ANSI Metric M Profile 5.0 M5x0.8 6H" major diameter 5.12 minor diameter 4.234 pitch 0.8 angle 60 resizes the face on face at (47.8837, 50.0528, 2.6667)
hole "Hole5" at (50, 30, 4) direction (0, 0, -1) diameter 4.234 depth 34 tip angle 180
thread "Thread5" "ANSI Metric M Profile 5.0 M5x0.8 6H" major diameter 5.12 minor diameter 4.234 pitch 0.8 angle 60 resizes the face on face at (50.2108, 32.1065, 2.6667)
hole "Hole6" at (30, 10, 4) direction (0, 0, -1) diameter 4.234 depth 34 tip angle 180
thread "Thread6" "ANSI Metric M Profile 5.0 M5x0.8 6H" major diameter 5.12 minor diameter 4.234 pitch 0.8 angle 60 resizes the face on face at (30.2108, 7.8935, 2.6667)

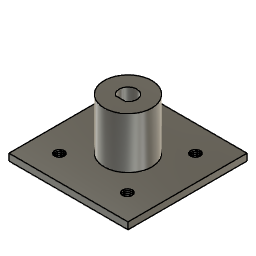
design "chamber_motor_mount"
Autodesk Fusion 360 part; units mm, degrees
sketch "Sketch1" plane through (0, 0, 0) normal (0, 0, 1) x (1, 0, 0)
  line L0 (0, 0) -> (35, 0)
  line L1 (35, 0) -> (35, 35)
  line L2 (35, 35) -> (0, 35)
  line L3 (0, 35) -> (0, 0)
  dimension "d1" = 35
  dimension "d2" = 35
  constraint horizontal L0
  constraint vertical L1
  constraint horizontal L2
  constraint vertical L3
  constraint coincident L0.start L3.end
  measures "d1" distance of L0.start L0.end
  measures "d2" distance of L0.start L2.end
extrude "Extrude1" add sketch "Sketch1" along normal blind 2
sketch "Sketch2" plane through (0, 0, 2) normal (0, 0, 1) x (-1, 0, 0)
  line L0 (0, -35) -> (0, 0)
  line L1 (0, 0) -> (-35, 0)
  line L2 (-35, 0) -> (-35, -35)
  line L3 (-35, -35) -> (0, -35)
  circle A0 centre (-7.5, -27.5) radius 1.5
  circle A1 centre (-27.5, -27.5) radius 1.5
  circle A2 centre (-7.5, -7.5) radius 1.5
  circle A3 centre (-27.5, -7.5) radius 1.5
  dimension "d6" = 3
  dimension "d7" = 3
  dimension "d8" = 3
  dimension "d9" = 3
  dimension "d30" = 20
  dimension "d31" = 20
  dimension "d32" = 20
  dimension "d33" = 20
  dimension "d34" = 7.5
  dimension "d35" = 7.5
  measures "d6" diameter of A0
  measures "d7" diameter of A1
  measures "d8" diameter of A2
  measures "d9" diameter of A3
  measures "d30" distance of A0.centre A1.centre
  measures "d31" distance of A2.centre A3.centre
  measures "d32" distance of A0.centre A2.centre
  measures "d33" distance of A1.centre A3.centre
  measures "d34" distance of L0 A0.centre
  measures "d35" distance of L1 A2.centre
hole "Hole1" at (7.5, 27.5, 2) at (27.5, 27.5, 2) at (27.5, 7.5, 2) at (7.5, 7.5, 2) direction (0, 0, -1) diameter 2.529 depth 2 tip angle 118
thread "Thread1" "ISO Metric profile 3.0 M3x0.5 M3x0.5 6H" major diameter 3.086 minor diameter 2.529 pitch 0.5 angle 60 modelled right hand crest width 0.1368 on face at (27.6259, 6.2418, 1.3333) crest through (28.7645, 7.5, 1.875) on face at (7.6259, 26.2418, 1.3333) crest through (8.7645, 27.5, 1.875) on face at (7.6259, 6.2418, 1.3333) crest through (8.7645, 7.5, 1.875) on face at (27.6259, 26.2418, 1.3333) crest through (28.7645, 27.5, 1.875)
sketch "Sketch3" plane through (0, 0, 2) normal (0, 0, 1) x (-1, 0, 0)
  spline S0 degree 3 poles (-28.4581, -8.3252) (-28.5802, -8.2112) (-28.6784, -8.074) (-28.8207, -7.764) (-28.8611, -7.593) (-28.8757, -7.2382) (-28.8471, -7.0577) (-28.7212, -6.7109) (-28.6226, -6.5488) (-28.4156, -6.3208) (-28.3244, -6.2423) (-28.1232, -6.1071) (-28.0136, -6.0514) (-27.8985, -6.0094) knots 0 0 0 0 0.050111 0.050111 0.102261 0.102261 0.15645 0.15645 0.212677 0.212677 0.24852 0.24852 0.285143 0.285143 0.285143 0.285143
  arc A0 (-27.1015, -6.0094) -> (-27.8985, -6.0094) centre (-27.5, -7.5) ccw
  spline S1 degree 3 poles (-27.1015, -6.0094) (-26.9166, -6.0769) (-26.7465, -6.1793) (-26.4611, -6.4399) (-26.3468, -6.5935) (-26.1876, -6.9304) (-26.1419, -7.1092) (-26.1233, -7.4674) (-26.148, -7.6432) (-26.241, -7.9082) (-26.2875, -8.0028) (-26.401, -8.1765) (-26.467, -8.2553) (-26.5419, -8.3252) knots 0 0 0 0 0.059039 0.059039 0.116033 0.116033 0.170983 0.170983 0.223888 0.223888 0.255505 0.255505 0.286347 0.286347 0.286347 0.286347
  arc A1 (-28.4581, -8.3252) -> (-26.5419, -8.3252) centre (-27.5, -7.5) ccw
  spline S2 degree 3 poles (-8.4581, -28.3252) (-8.5802, -28.2112) (-8.6784, -28.074) (-8.8207, -27.764) (-8.8611, -27.593) (-8.8757, -27.2382) (-8.8471, -27.0577) (-8.7212, -26.7109) (-8.6226, -26.5488) (-8.4156, -26.3208) (-8.3244, -26.2423) (-8.1232, -26.1071) (-8.0136, -26.0514) (-7.8985, -26.0094) knots 0 0 0 0 0.050111 0.050111 0.102261 0.102261 0.15645 0.15645 0.212677 0.212677 0.24852 0.24852 0.285143 0.285143 0.285143 0.285143
  arc A2 (-7.1015, -26.0094) -> (-7.8985, -26.0094) centre (-7.5, -27.5) ccw
  spline S3 degree 3 poles (-7.1015, -26.0094) (-6.9166, -26.0769) (-6.7465, -26.1793) (-6.4611, -26.4399) (-6.3468, -26.5935) (-6.1876, -26.9304) (-6.1419, -27.1092) (-6.1233, -27.4674) (-6.148, -27.6432) (-6.241, -27.9082) (-6.2875, -28.0028) (-6.401, -28.1765) (-6.467, -28.2553) (-6.5419, -28.3252) knots 0 0 0 0 0.059039 0.059039 0.116033 0.116033 0.170983 0.170983 0.223888 0.223888 0.255505 0.255505 0.286347 0.286347 0.286347 0.286347
  arc A3 (-8.4581, -28.3252) -> (-6.5419, -28.3252) centre (-7.5, -27.5) ccw
  spline S4 degree 3 poles (-28.4581, -28.3252) (-28.5802, -28.2112) (-28.6784, -28.074) (-28.8207, -27.764) (-28.8611, -27.593) (-28.8757, -27.2382) (-28.8471, -27.0577) (-28.7212, -26.7109) (-28.6226, -26.5488) (-28.4156, -26.3208) (-28.3244, -26.2423) (-28.1232, -26.1071) (-28.0136, -26.0514) (-27.8985, -26.0094) knots 0 0 0 0 0.050111 0.050111 0.102261 0.102261 0.15645 0.15645 0.212677 0.212677 0.24852 0.24852 0.285143 0.285143 0.285143 0.285143
  arc A4 (-27.1015, -26.0094) -> (-27.8985, -26.0094) centre (-27.5, -27.5) ccw
  spline S5 degree 3 poles (-27.1015, -26.0094) (-26.9166, -26.0769) (-26.7465, -26.1793) (-26.4611, -26.4399) (-26.3468, -26.5935) (-26.1876, -26.9304) (-26.1419, -27.1092) (-26.1233, -27.4674) (-26.148, -27.6432) (-26.241, -27.9082) (-26.2875, -28.0028) (-26.401, -28.1765) (-26.467, -28.2553) (-26.5419, -28.3252) knots 0 0 0 0 0.059039 0.059039 0.116033 0.116033 0.170983 0.170983 0.223888 0.223888 0.255505 0.255505 0.286347 0.286347 0.286347 0.286347
  arc A5 (-28.4581, -28.3252) -> (-26.5419, -28.3252) centre (-27.5, -27.5) ccw
  spline S6 degree 3 poles (-8.4581, -8.3252) (-8.5802, -8.2112) (-8.6784, -8.074) (-8.8207, -7.764) (-8.8611, -7.593) (-8.8757, -7.2382) (-8.8471, -7.0577) (-8.7212, -6.7109) (-8.6226, -6.5488) (-8.4156, -6.3208) (-8.3244, -6.2423) (-8.1232, -6.1071) (-8.0136, -6.0514) (-7.8985, -6.0094) knots 0 0 0 0 0.050111 0.050111 0.102261 0.102261 0.15645 0.15645 0.212677 0.212677 0.24852 0.24852 0.285143 0.285143 0.285143 0.285143
  arc A6 (-7.1015, -6.0094) -> (-7.8985, -6.0094) centre (-7.5, -7.5) ccw
  spline S7 degree 3 poles (-7.1015, -6.0094) (-6.9166, -6.0769) (-6.7465, -6.1793) (-6.4611, -6.4399) (-6.3468, -6.5935) (-6.1876, -6.9304) (-6.1419, -7.1092) (-6.1233, -7.4674) (-6.148, -7.6432) (-6.241, -7.9082) (-6.2875, -8.0028) (-6.401, -8.1765) (-6.467, -8.2553) (-6.5419, -8.3252) knots 0 0 0 0 0.059039 0.059039 0.116033 0.116033 0.170983 0.170983 0.223888 0.223888 0.255505 0.255505 0.286347 0.286347 0.286347 0.286347
  arc A7 (-8.4581, -8.3252) -> (-6.5419, -8.3252) centre (-7.5, -7.5) ccw
  line L0 (0, -35) -> (0, 0)
  line L1 (0, 0) -> (-35, 0)
  line L2 (-35, 0) -> (-35, -35)
  line L3 (-35, -35) -> (0, -35)
  circle A8 centre (-17.5, -17.5) radius 12
  dimension "d15" = 24
  dimension "d16" = 17.5
  dimension "d17" = 17.5
  measures "d15" diameter of A8
  measures "d16" distance of L2 A8.centre
  measures "d17" distance of L3 A8.centre
extrude "Extrude2" add sketch "Sketch3" along normal blind 20 contours A8
sketch "Sketch4" plane through (0, 0, 22) normal (0, 0, 1) x (-1, 0, 0)
  circle A0 centre (-17.5, -17.5) radius 12
  circle A1 centre (-17.5, -17.5) radius 7
  dimension "d20" = 14
  constraint concentric A0 A1
  measures "d20" diameter of A1
extrude "Extrude3" add sketch "Sketch4" along normal blind 20 contours A1
sketch "Sketch5" plane through (0, 0, 42) normal (0, 0, 1) x (-1, 0, 0)
  circle A0 centre (-17.5, -17.5) radius 7
  line L0 (-16.0593, -15.3057) -> (-18.9407, -15.3057)
  arc A1 (-18.9407, -15.3057) -> (-16.0593, -15.3057) centre (-17.5, -17.5) ccw
  dimension "d23" = 5.25
  constraint concentric A0 A1
  constraint horizontal L0
  measures "d23" diameter of A1
extrude "Extrude4" cut sketch "Sketch5" against normal blind 39 contours L0 A1
extrude "Extrude5" cut 1 faces at (7.2113, 18.0962, 22) along direction (0, 0, -1) blind 20
extrude "Extrude6" cut 1 faces at (17.3256, 13.7103, 42) along direction (0, 0, -1) blind 25
